Support Button (Autodesk Fusion 360 design; units mm, degrees)
Autodesk Fusion 360 part; units mm, degrees
note: some values were not read from the file. Set by a fixed rule: which sketch regions a step uses.
sketch "Sketch2" plane through (0, 0, 0) normal (1, 0, 0) x (0, 1, 0) in component "Support Batt"
  circle A0 centre (154.2359, 79.3135) radius 4
  line L0 (99.2359, 44.7135) -> (119.2359, 44.7135)
  line L1 (119.2359, 31.7135) -> (119.2359, 44.7135)
  line L2 (99.2359, 31.7135) -> (99.2359, 44.7135)
  line L3 (160.5859, 85.8135) -> (106.4359, 85.8135)
  line L4 (50.5431, 31.7135) -> (52.3447, 31.7135)
  line L5 (52.3447, 31.7135) -> (217.041, 31.7135) construction
  line L6 (96.4359, 75.8135) -> (96.4359, 31.7135)
  line L7 (96.4359, 31.7135) -> (98.9359, 31.7135)
  line L8 (98.9359, 44.7135) -> (119.5359, 44.7135)
  line L9 (119.5359, 44.7135) -> (119.5359, 31.7135)
  line L10 (98.9359, 44.7135) -> (98.9359, 31.7135)
  line L11 (119.5359, 31.7135) -> (122.0359, 31.7135)
  line L12 (154.2359, 83.3135) -> (160.5859, 83.3135) construction
  line L13 (160.5859, 85.8135) -> (160.5859, 70.8135)
  line L14 (158.0859, 70.8135) -> (160.5859, 70.8135)
  line L15 (158.0859, 78.2283) -> (158.0859, 70.8135)
  line L16 (150.3859, 78.2283) -> (150.3859, 70.8135)
  line L17 (150.3859, 70.8135) -> (147.8859, 70.8135)
  line L18 (150.3859, 70.8135) -> (158.0859, 70.8135) construction
  line L19 (154.2359, 79.3135) -> (154.2359, 70.8135) construction
  line L20 (147.8859, 70.8135) -> (147.8859, 71.8135)
  line L21 (137.8859, 81.8135) -> (110.4359, 81.8135)
  line L22 (122.0359, 31.7135) -> (122.0359, 47.7135)
  line L23 (122.0359, 47.7135) -> (110.4359, 47.7135)
  line L24 (100.4359, 57.7135) -> (100.4359, 71.8135)
  arc A1 (110.4359, 81.8135) -> (100.4359, 71.8135) centre (110.4359, 71.8135) ccw
  arc A2 (147.8859, 71.8135) -> (137.8859, 81.8135) centre (137.8859, 71.8135) ccw
  arc A3 (100.4359, 57.7135) -> (110.4359, 47.7135) centre (110.4359, 57.7135) ccw
  arc A4 (158.0859, 78.2283) -> (150.3859, 78.2283) centre (154.2359, 79.3135) ccw
  arc A5 (106.4359, 85.8135) -> (96.4359, 75.8135) centre (106.4359, 75.8135) ccw
  line L25 (114.8859, 81.8135) -> (117.8859, 81.8135)
  line L26 (117.8859, 81.8135) -> (117.8859, 78.8135)
  line L27 (117.8859, 78.8135) -> (114.8859, 78.8135)
  line L28 (114.8859, 78.8135) -> (114.8859, 81.8135)
  line L29 (160.5859, 85.8135) -> (185.5859, 85.8135)
  line L30 (185.5859, 85.8135) -> (185.5859, 82.8135)
  line L31 (185.5859, 82.8135) -> (160.5859, 82.8135)
  line L32 (160.5859, 82.8135) -> (160.5859, 85.8135)
  line L33 (160.5859, 70.8135) -> (185.5859, 82.8135)
  point P0 (96.4359, 85.8135)
  point P1 (100.4359, 81.8135)
  dimension "d2" = 0.3
  dimension "d3" = 0.3
  dimension "d4" = 2.5
  dimension "d5" = 2.5
  dimension "d6" = 2.5
  dimension "d7" = 2.5
  dimension "d8" = 8
  dimension "d9" = 15
  dimension "d10" = 7.7
  dimension "d11" = 2.5
  dimension "d12" = 4
  dimension "d13" = 4
  dimension "d14" = 3
  dimension "d15" = 10
  dimension "d68" = 10
  dimension "d69" = 3
  dimension "d70" = 3
  dimension "d71" = 30
  dimension "d80" = 25
  dimension "d81" = 3
  constraint horizontal L3
  constraint horizontal L4
  constraint parallel L4 L5
  constraint coincident L2.start L5
  constraint coincident L5 L6.end
  constraint perpendicular L5 L6
  constraint coincident L5 L7.end
  constraint perpendicular L6 L8
  constraint coincident L5 L9.end
  constraint perpendicular L8 L9
  constraint perpendicular L7 L10
  constraint coincident L0.start L8
  constraint coincident L5 L11.end
  constraint parallel L3 L12
  constraint vertical L13
  constraint horizontal L14
  constraint concentric A0 A4
  constraint coincident A0 L15.start
  constraint vertical L15
  constraint coincident A0 L16.start
  constraint vertical L16
  constraint perpendicular L16 L17
  constraint horizontal L18
  constraint coincident A0.centre L19.start
  constraint midpoint L18 L19.end
  constraint vertical L19
  constraint tangent L12 A4
  constraint perpendicular L17 L20
  constraint perpendicular L20 L21
  constraint coincident A0 L12.start
  constraint perpendicular L11 L22
  constraint perpendicular L22 L23
  constraint vertical L24
  constraint coincident P1 L21
  constraint coincident P1 L24
  constraint tangent L21 A1
  constraint tangent L24 A1
  constraint tangent L21 A2
  constraint tangent L20 A2
  constraint equal A1 A2
  constraint tangent L23 A3
  constraint tangent L24 A3
  constraint equal A1 A3
  constraint coincident P0 L6
  constraint coincident P0 L3
  constraint tangent L3 A5
  constraint tangent L6 A5
  constraint horizontal L25
  constraint vertical L26
  constraint horizontal L27
  constraint vertical L28
  constraint coincident L21 L25.start
  constraint horizontal L29
  constraint vertical L30
  constraint horizontal L31
  constraint vertical L32
  measures "d2" distance of L2.start L7.end
  measures "d3" distance of L1.start L9.end
  measures "d4" distance of L6.end L7.end
  measures "d5" distance of L9.end L11.end
  measures "d6" distance of L3 L12
  measures "d7" distance of L13.end L14.start
  measures "d8" diameter of A4
  measures "d9" distance of L3.start L13.end
  measures "d10" distance of L14.start L16.end
  measures "d11" distance of L16 L20
  measures "d12" distance of L3 L21
  measures "d13" horizontal distance of P0 P1
  measures "d14" vertical distance of L8.end L22.end
  measures "d15" radius of A1
  measures "d68" radius of A5
  measures "d69" distance of L26.end L27.end
  measures "d70" distance of L25.start L27.end
  measures "d71" horizontal distance of L17.end L26.end
  measures "d80" distance of L3.start L29.end
  measures "d81" distance of L3.start L31.end
extrude "Extrude1" add sketch "Sketch2" along normal blind 40 contours A0 L0 L3 L6 L7 L8 L9 L10 L11 L13 L14 L15 L16 L17 L20 L21 L22 L23 L24 A1 A2 A3 A4 A5 L25 L32 | L13 L29 L30 L31 L32 | L21 L25 L26 L27 L28 in component "Support Batt"
sketch "Sketch3" plane through (0, 0, 44.7135) normal (0, 0, -1) x (1, 0, 0) in component "Support Batt"
  line L0 (0, -98.9359) -> (0, -119.5359)
  line L1 (0, -119.5359) -> (40, -119.5359)
  line L2 (40, -119.5359) -> (40, -98.9359)
  line L3 (40, -98.9359) -> (0, -98.9359)
  line L4 (0, -109.2359) -> (40, -109.2359) construction
  circle A0 centre (25, -109.2359) radius 1.6
  circle A1 centre (15, -109.2359) radius 1.6
  line L5 (15, -109.2359) -> (25, -109.2359)
  line L6 (20, -109.2359) -> (20, -98.9359)
  circle A2 centre (35, -109.2359) radius 1.6
  circle A3 centre (5, -109.2359) radius 1.6
  dimension "d18" = 3.2
  dimension "d19" = 3.2
  dimension "d33" = 3.2
  dimension "d34" = 3.2
  dimension "d35" = 10
  dimension "d36" = 10
  dimension "d72" = 10
  constraint midpoint L0 L4.start
  constraint midpoint L2 L4.end
  constraint coincident L4 A0.centre
  constraint coincident L4 A1.centre
  constraint coincident A1.centre L5.start
  constraint coincident A0.centre L5.end
  constraint midpoint L5 L6.start
  constraint midpoint L3 L6.end
  constraint vertical L6
  constraint coincident L4 A2.centre
  constraint coincident L4 A3.centre
  measures "d18" diameter of A0
  measures "d19" diameter of A1
  measures "d33" diameter of A2
  measures "d34" diameter of A3
  measures "d35" distance of A1.centre A3.centre
  measures "d36" distance of A0.centre A2.centre
  measures "d72" distance of A0.centre A1.centre
extrude "Extrude2" cut sketch "Sketch3" against normal blind 17 contours A0 | A1 | A2 | A3 in component "Support Batt"
sketch "Sketch4" plane through (0, 0, 47.7135) normal (0, 0, 1) x (-1, 0, 0) in component "Support Batt"
  arc A0 (-26.0583, -110.4359) -> (-23.9417, -110.4359) centre (-25, -109.2359) ccw
  line L0 (-26.0583, -110.4359) -> (-33.9417, -110.4359)
  line L1 (-40, -110.4359) -> (-40, -122.0359)
  line L2 (-40, -122.0359) -> (0, -122.0359)
  line L3 (0, -122.0359) -> (0, -110.4359)
  line L4 (0, -110.4359) -> (-3.9417, -110.4359)
  arc A1 (-16.0583, -110.4359) -> (-13.9417, -110.4359) centre (-15, -109.2359) ccw
  line L5 (-16.0583, -110.4359) -> (-23.9417, -110.4359)
  circle A2 centre (-15, -109.2359) radius 3.25
  circle A3 centre (-25, -109.2359) radius 3.25
  arc A4 (-36.0583, -110.4359) -> (-33.9417, -110.4359) centre (-35, -109.2359) ccw
  line L6 (-36.0583, -110.4359) -> (-40, -110.4359)
  arc A5 (-6.0583, -110.4359) -> (-3.9417, -110.4359) centre (-5, -109.2359) ccw
  line L7 (-6.0583, -110.4359) -> (-13.9417, -110.4359)
  circle A6 centre (-5, -109.2359) radius 3.25
  circle A7 centre (-35, -109.2359) radius 3.25
  dimension "d22" = 6.5
  dimension "d23" = 6.5
  dimension "d37" = 6.5
  dimension "d38" = 6.5
  constraint concentric A1 A2
  constraint concentric A0 A3
  constraint concentric A5 A6
  constraint concentric A4 A7
  measures "d22" diameter of A2
  measures "d23" diameter of A3
  measures "d37" diameter of A6
  measures "d38" diameter of A7
extrude "Extrude3" cut sketch "Sketch4" along normal blind 1.0447 contours A0 L0 L5 A3 | L0 A4 L6 A7 | A1 L5 A2 L7 | L4 A5 L7 A6 picked at (-25.046, -108.9536) picked at (-35.046, -108.9536) picked at (-15.046, -108.9536) picked at (-5.046, -108.9536) in component "Support Batt"
extrude "Extrude3'" add sketch "Sketch2" along normal blind 4 contours L13 L31 L33 in component "Support Batt"
sketch "Sketch5" plane through (40, 0, 0) normal (1, 0, 0) x (0, 1, 0) in component "Support Batt"
  line L0 (158.0859, 70.8135) -> (160.5859, 70.8135)
  line L1 (160.5859, 70.8135) -> (160.5859, 82.8135)
  line L2 (160.5859, 82.8135) -> (185.5859, 82.8135)
  line L3 (185.5859, 82.8135) -> (185.5859, 85.8135)
  line L4 (185.5859, 85.8135) -> (106.4359, 85.8135)
  arc A0 (106.4359, 85.8135) -> (96.4359, 75.8135) centre (106.4359, 75.8135) ccw
  line L5 (96.4359, 75.8135) -> (96.4359, 31.7135)
  line L6 (96.4359, 31.7135) -> (98.9359, 31.7135)
  line L7 (98.9359, 31.7135) -> (98.9359, 44.7135)
  line L8 (98.9359, 44.7135) -> (119.5359, 44.7135)
  line L9 (119.5359, 44.7135) -> (119.5359, 31.7135)
  line L10 (119.5359, 31.7135) -> (122.0359, 31.7135)
  line L11 (122.0359, 31.7135) -> (122.0359, 47.7135)
  line L12 (122.0359, 47.7135) -> (110.4359, 47.7135)
  arc A1 (100.4359, 57.7135) -> (110.4359, 47.7135) centre (110.4359, 57.7135) ccw
  line L13 (100.4359, 57.7135) -> (100.4359, 71.8135)
  arc A2 (110.4359, 81.8135) -> (100.4359, 71.8135) centre (110.4359, 71.8135) ccw
  line L14 (110.4359, 81.8135) -> (114.8859, 81.8135)
  line L15 (114.8859, 81.8135) -> (114.8859, 78.8135)
  line L16 (114.8859, 78.8135) -> (117.8859, 78.8135)
  line L17 (117.8859, 78.8135) -> (117.8859, 81.8135)
  line L18 (117.8859, 81.8135) -> (137.8859, 81.8135)
  arc A3 (147.8859, 71.8135) -> (137.8859, 81.8135) centre (137.8859, 71.8135) ccw
  line L19 (147.8859, 71.8135) -> (147.8859, 70.8135)
  line L20 (147.8859, 70.8135) -> (150.3859, 70.8135)
  line L21 (150.3859, 70.8135) -> (150.3859, 78.2283)
  arc A4 (158.0859, 78.2283) -> (150.3859, 78.2283) centre (154.2359, 79.3135) ccw
  line L22 (158.0859, 78.2283) -> (158.0859, 70.8135)
  line L23 (160.5859, 70.8135) -> (185.5859, 82.8135)
  constraint coincident L0.end L1.start
  constraint coincident L2.end L3.start
extrude "Extrude4" add sketch "Sketch5" against normal blind 4 contours L1 L2 L23 in component "Support Batt"
sketch "Sketch4 (1)" plane through (0, 0, 81.8135) normal (0, 0, -1) x (1, 0, 0) in component "Support Batt"
  line L0 (0, -117.8859) -> (0, -137.8859)
  line L1 (0, -137.8859) -> (40, -137.8859)
  line L2 (40, -137.8859) -> (40, -117.8859)
  line L3 (40, -117.8859) -> (0, -117.8859)
  line L4 (0, -147.8859) -> (40, -147.8859)
  line L5 (40, -147.8859) -> (0, -117.8859) construction
  line L6 (0, -158.0859) -> (0, -160.5859) construction
  line L7 (0, -160.5859) -> (4, -160.5859) construction
  line L8 (4, -160.5859) -> (36, -160.5859) construction
  line L9 (36, -160.5859) -> (40, -160.5859) construction
  line L10 (40, -160.5859) -> (40, -158.0859) construction
  line L11 (40, -158.0859) -> (0, -158.0859) construction
  line L12 (0, -160.5859) -> (0, -185.5859) construction
  line L13 (0, -185.5859) -> (4, -185.5859) construction
  line L14 (4, -185.5859) -> (4, -160.5859) construction
  line L15 (4, -160.5859) -> (0, -160.5859) construction
  circle A0 centre (20, -172.0859) radius 10.5
  circle A1 centre (20, -132.8859) radius 11
  line L16 (1.5, -147.8859) -> (38.5, -147.8859)
  line L17 (38.5, -147.8859) -> (38.5, -117.8859)
  line L18 (38.5, -117.8859) -> (1.5, -117.8859)
  line L19 (1.5, -117.8859) -> (1.5, -147.8859)
  line L20 (1.5, -147.8859) -> (38.5, -117.8859) construction
  line L21 (38.5, -147.8859) -> (1.5, -117.8859) construction
  line L22 (20, -158.0859) -> (20, -172.0859)
  point P0 (20, -132.8859)
  dimension "d88" = 21
  dimension "d89" = 22
  dimension "d90" = 37
  dimension "d91" = 30
  dimension "d96" = 14
  constraint coincident L4.end L5.start
  constraint coincident L0.start L3.end
  constraint midpoint L5 P0
  constraint horizontal L16
  constraint perpendicular L16 L17
  constraint parallel L16 L18
  constraint parallel L17 L19
  constraint coincident L20 P0
  constraint coincident L21 P0
  constraint coincident P0 A1.centre
  constraint midpoint L11 L22.start
  constraint coincident A0.centre L22.end
  constraint perpendicular L8 L22
  measures "d88" diameter of A0
  measures "d89" diameter of A1
  measures "d90" distance of L17.end L18.end
  measures "d91" distance of L16.end L17.end
  measures "d96" distance of L22.start A0.centre
extrude "Extrude5" cut sketch "Sketch4 (1)" against normal blind 11 contours L1 A1 | L1 A1 | A0 in component "Support Batt"
extrude "Extrude6" cut sketch "Sketch4 (1)" along normal blind 17 contours L1 L4 A1 L16 L17 L19 | L1 A1 picked at (22.1414, -140.7456) in component "Support Batt"
component "Support Batt" placed x (1, 0, 0) y (0, 1, 0) z (0, 0, 1) at (0, 0, 0)
named bodies: "Support_Button"
